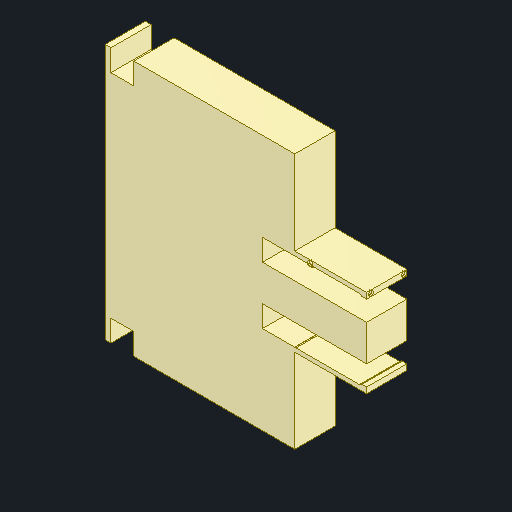
# Autodesk Inventor part: right_hold
Saved by Autodesk Inventor 2023 (Build 270158000, 158)
## iProperties
Created: 2024-05-18
Part Number: right_hold
Material: Nylon 6/6
Document SubType Name: Modeling
Designer: szymo
Density: 1.13 g/cm^3
Appearance: Nylon 6
Mass: 756.104 g
Surface Area: 779.57 cm^2
Volume: 669.119 cm^3
Author: szymo
Autodesk Inventor part; units mm, degrees
(part 1 of 2)
ref_plane "YZ Plane" through (0, 0, 0) normal (1, 0, 0) x (0, 1, 0)
ref_plane "XZ Plane" through (0, 0, 0) normal (0, 1, 0) x (-1, 0, 0)
ref_plane "XY Plane" through (0, 0, 0) normal (0, 0, 1) x (1, 0, 0)
ref_plane "Work Plane1" through (0, 0, 0) normal (0, 0, 1) x (1, 0, 0)
sketch "Sketch1" plane through (0, 0, 0) normal (0, 0, 1) x (1, 0, 0)
  line L0 (-71, -74) -> (-71, -89) projected
  line L1 (-71, -89) -> (41, -89) projected
  line L2 (41, -89) -> (41, -30.5) projected
  line L3 (41, -30.5) -> (91, -30.5) projected
  line L4 (91, -30.5) -> (91, -26.5) projected
  line L5 (91, 30.5) -> (41, 30.5) projected
  line L6 (41, 30.5) -> (41, 89) projected
  line L7 (41, 89) -> (-71, 89) projected
  line L8 (-71, 89) -> (-71, 74) projected
  line L9 (-71, 74) -> (-87, 74) projected
  line L10 (-87, 74) -> (-87, 89) projected
  line L11 (-87, 89) -> (-91, 89) projected
  line L12 (-91, 89) -> (-91, -89) projected
  line L13 (-91, -89) -> (-87, -89) projected
  line L14 (-87, -89) -> (-87, -74) projected
  line L15 (-87, -74) -> (-71, -74) projected
  line L16 (91, 30.5) -> (12, 30.5)
  line L17 (12, 30.5) -> (12, 29.5)
  line L18 (12, 29.5) -> (91, 29.5)
  line L19 (91, 29.5) -> (91, 30.5)
  line L20 (71.5, 26) -> (60.5, 26) projected
  line L21 (11.5, 37) -> (39.5, 37) projected
  line L22 (11, 8.5) -> (11, 9.5)
  circle A0 centre (15.25, 24.25) radius 1.8 projected
  circle A1 centre (15.25, -15.75) radius 1.8 projected
  circle A2 centre (6.1414, -28.5) radius 1.8 projected
  circle A3 centre (-23.4, 24.1) radius 1.8 projected
  circle A4 centre (-71.6, -24.1) radius 1.8 projected
  circle A5 centre (-82.75, 33.75) radius 1.8 projected
  circle A6 centre (-67.5, -84.5) radius 1.8 projected
  circle A7 centre (88, -10.5) radius 1.8 projected
  circle A8 centre (88, 10.5) radius 1.8 projected
  circle A9 centre (-67.5, 84.5) radius 1.8 projected
  circle A10 centre (-71.6, 24.1) radius 1.8 projected
  circle A11 centre (-82.75, -33.75) radius 1.8 projected
  circle A12 centre (-23.4, -24.1) radius 1.8 projected
  circle A13 centre (15.25, -24.25) radius 1.8 projected
  circle A14 centre (15.25, 15.75) radius 1.8 projected
  circle A15 centre (6.1414, 28.5) radius 1.8 projected
  circle A16 centre (-51.4385, -83.5) radius 1.55 projected
  circle A17 centre (-24.4119, -29.75) radius 1.55 projected
  circle A18 centre (-49.009, 29.75) radius 1.55 projected
  circle A19 centre (-22.5, 83.5) radius 1.55 projected
  circle A20 centre (8.5, -82.4087) radius 1.55 projected
  circle A21 centre (8.5, 82.4087) radius 1.55 projected
  circle A22 centre (-51.4385, 83.5) radius 1.55 projected
  circle A23 centre (-24.4119, 29.75) radius 1.55 projected
  circle A24 centre (-49.009, -29.75) radius 1.55 projected
  circle A25 centre (-22.5, -83.5) radius 1.55 projected
  circle A26 centre (-83, 21.5) radius 1.8 projected
  circle A27 centre (-83, -64.5) radius 1.8 projected
  circle A28 centre (-83, -21.5) radius 1.8 projected
  circle A29 centre (-83, 64.5) radius 1.8 projected
  line L23 (87.7321, 26.5) -> (91, 26.5) projected
  line L24 (91, 26.5) -> (91, 30.5) projected
  line L25 (91, -26.5) -> (87.7321, -26.5) projected
  arc A30 (87.7321, -26.5) -> (86.866, -27) centre (87.7321, -27.5) ccw projected
  arc A31 (86, -27.5) -> (86.866, -27) centre (86, -26.5) ccw projected
  line L26 (86, -27.5) -> (41.8217, -27.5) projected
  ellipse E0 centre (41.4293, -27.1664) end of major axis (40.558, -26.9979) minor radius 0.2933 (41, -27.3523) -> (41.8217, -27.5) ccw projected
  line L27 (41, -27.3523) -> (41, -27.5) projected
  line L28 (41, -27.5) -> (18.5, -27.5) projected
  line L29 (18.5, -27.5) -> (18.5, -12.5) projected
  line L30 (18.5, -12.5) -> (91, -12.5) projected
  line L31 (91, -12.5) -> (91, 12.5) projected
  line L32 (91, 12.5) -> (18.5, 12.5) projected
  line L33 (18.5, 12.5) -> (18.5, 27.5) projected
  line L34 (18.5, 27.5) -> (41, 27.5) projected
  line L35 (41, 27.5) -> (41, 27.3523) projected
  ellipse E1 centre (41.4293, 27.1664) end of major axis (40.558, 26.9979) minor radius 0.2933 (41.8217, 27.5) -> (41, 27.3523) ccw projected
  line L36 (41.8217, 27.5) -> (86, 27.5) projected
  arc A32 (86.866, 27) -> (86, 27.5) centre (86, 26.5) ccw projected
  arc A33 (86.866, 27) -> (87.7321, 26.5) centre (87.7321, 27.5) ccw projected
  line L37 (-85, 14) -> (-76, 14) projected
  line L38 (-76, 14) -> (-76, 20.1) projected
  line L39 (-76, 20.1) -> (11.5, 20.1) projected
  line L40 (11.5, 20.1) -> (11.5, 8.5) projected
  line L41 (11.5, 8.5) -> (84, 8.5) projected
  line L42 (84, 8.5) -> (84, -8.5) projected
  line L43 (84, -8.5) -> (11.5, -8.5) projected
  line L44 (11.5, -8.5) -> (11.5, -20.1) projected
  line L45 (11.5, -20.1) -> (-76, -20.1) projected
  line L46 (-76, -20.1) -> (-76, -14) projected
  line L47 (-76, -14) -> (-85, -14) projected
  arc A34 (-87, -12) -> (-85, -14) centre (-85, -12) ccw projected
  line L48 (-87, -12) -> (-87, 12) projected
  arc A35 (-85, 14) -> (-87, 12) centre (-85, 12) ccw projected
  line L49 (-76, 57) -> (-64, 69) projected
  line L50 (-64, 69) -> (-64, 79.9087) projected
  line L51 (-64, 79.9087) -> (15.1148, 79.9087) projected
  line L52 (15.1148, 79.9087) -> (15.1148, 37) projected
  line L53 (15.1148, 37) -> (-86, 37) projected
  line L54 (-86, 37) -> (-86, 29.2679) projected
  arc A36 (-87, 31) -> (-86, 29.2679) centre (-85, 31) ccw projected
  line L55 (-87, 31) -> (-87, 55) projected
  arc A37 (-85, 57) -> (-87, 55) centre (-85, 55) ccw projected
  line L56 (-85, 57) -> (-76, 57) projected
  line L57 (-64, -79.9087) -> (-64, -69) projected
  line L58 (-64, -69) -> (-76, -57) projected
  line L59 (-76, -57) -> (-85, -57) projected
  arc A38 (-87, -55) -> (-85, -57) centre (-85, -55) ccw projected
  line L60 (-87, -55) -> (-87, -37) projected
  line L61 (-87, -37) -> (15.1148, -37) projected
  line L62 (15.1148, -37) -> (15.1148, -79.9087) projected
  line L63 (15.1148, -79.9087) -> (-64, -79.9087) projected
  line L64 (30.8852, 37) -> (20.1148, 37) projected
  line L65 (20.1148, 37) -> (20.1148, 79.9087) projected
  line L66 (20.1148, 79.9087) -> (30.8852, 79.9087) projected
  line L67 (30.8852, 79.9087) -> (30.8852, 37) projected
  line L68 (30.8852, -79.9087) -> (20.1148, -79.9087) projected
  line L69 (20.1148, -79.9087) -> (20.1148, -37) projected
  line L70 (20.1148, -37) -> (30.8852, -37) projected
  line L71 (30.8852, -37) -> (30.8852, -79.9087) projected
  point P0 (0, 0)
  dimension "d0" = 0
  dimension "d1" = 3.5
  dimension "d2" = 1
  dimension "d14" = 1
  constraints: 10 end point, 2 parallel, 1 horizontal, 1 perpendicular, 1 point on line, 1 vertical, 4 other
  measures "d0" distance between parallel lines of L5 L16
  measures "d1" distance between parallel lines of L18 L20
  measures "d2" distance between parallel lines of L16 L18
  measures "d14" distance between parallel lines of L22 L17
ref_plane "Work Plane2" through (11, 8.5, 30) normal (0, 0, 1) x (1, 0, 0)
extrude "Extrusion1" add sketch "Sketch1" along normal blind 28 contours L15 L14 L13 L12 L11 L10 L9 L8 L7 L6 L16 L17 L18 L24 L23 A33 A32 L36 E1 L35 L34 L33 L32 L31 L30 L29 L28 L27 E0 L26 A31 A30 L25 L4 L3 L2 L1 L0 | L5 L19 L18 L17 L16 | L53 L54 A36 L55 A37 L56 L49 L50 L51 L52 L21 | L65 L66 L67 L21 | A0 | A1 | A2 | A3 | A4 | A5 | A6 | A7 | A8 | A9 | A10 | A11 | A12 | A13 | A14 | A15 | A16 | A17 | A18 | A19 | A20 | A21 | A22 | A23 | A24 | A25 | A26 | A27 | A28 | A29 | L37 L38 L39 L40 L41 L42 L43 L44 L45 L46 L47 A34 L48 A35 | L57 L58 L59 A38 L60 L61 L62 L63 | L68 L69 L70 L71
sketch "Sketch2" plane through (12, 29.5, 0) normal (0, -1, 0) x (1, 0, 0)
  circle A0 centre (54, 6.5) radius 3.9
  arc A1 (11.0575, 16.9943) -> (9.1437, 17.8944) centre (8.1132, 13.2185) ccw projected
  arc A2 (9.1437, 17.8944) -> (8.5881, 17.165) centre (13.5, 14) ccw projected
  arc A3 (8.5881, 17.165) -> (9.9644, 15.5591) centre (12.822, 19.4008) ccw projected
  arc A4 (9.9644, 15.5591) -> (9.764, 14.9868) centre (13.5, 14) ccw projected
  arc A5 (9.764, 14.9868) -> (7.6866, 14.59) centre (9.6013, 10.2015) ccw projected
  arc A6 (7.6866, 14.59) -> (7.6659, 13.6734) centre (13.5, 14) ccw projected
  arc A7 (7.6659, 13.6734) -> (9.7232, 13.1831) centre (9.777, 17.9709) ccw projected
  arc A8 (9.7232, 13.1831) -> (9.8975, 12.6024) centre (13.5, 14) ccw projected
  arc A9 (9.8975, 12.6024) -> (8.45, 11.0603) centre (12.5786, 8.6353) ccw projected
  arc A10 (8.45, 11.0603) -> (8.9721, 10.3065) centre (13.5, 14) ccw projected
  arc A11 (8.9721, 10.3065) -> (10.9247, 11.1192) centre (8.154, 15.0242) ccw projected
  arc A12 (10.9247, 11.1192) -> (11.407, 10.7518) centre (13.5, 14) ccw projected
  arc A13 (11.407, 10.7518) -> (11.1424, 8.6535) centre (15.9078, 9.1183) ccw projected
  arc A14 (11.1424, 8.6535) -> (12.0078, 8.3505) centre (13.5, 14) ccw projected
  arc A15 (12.0078, 8.3505) -> (13.1098, 10.1556) centre (8.573, 11.6863) ccw projected
  arc A16 (13.1098, 10.1556) -> (13.716, 10.1419) centre (13.5, 14) ccw projected
  arc A17 (13.716, 10.1419) -> (14.7353, 8.2888) centre (18.3174, 11.4659) ccw projected
  arc A18 (14.7353, 8.2888) -> (15.6135, 8.5523) centre (13.5, 14) ccw projected
  arc A19 (15.6135, 8.5523) -> (15.444, 10.6605) centre (10.8739, 9.2321) ccw projected
  arc A20 (15.444, 10.6605) -> (15.9425, 11.0057) centre (13.5, 14) ccw projected
  arc A21 (15.9425, 11.0057) -> (17.8563, 10.1056) centre (18.8868, 14.7815) ccw projected
  arc A22 (17.8563, 10.1056) -> (18.4119, 10.835) centre (13.5, 14) ccw projected
  arc A23 (18.4119, 10.835) -> (17.0356, 12.4409) centre (14.178, 8.5992) ccw projected
  arc A24 (17.0356, 12.4409) -> (17.236, 13.0132) centre (13.5, 14) ccw projected
  arc A25 (17.236, 13.0132) -> (19.3134, 13.41) centre (17.3987, 17.7985) ccw projected
  arc A26 (19.3134, 13.41) -> (19.3341, 14.3266) centre (13.5, 14) ccw projected
  arc A27 (19.3341, 14.3266) -> (17.2768, 14.8169) centre (17.223, 10.0291) ccw projected
  arc A28 (17.2768, 14.8169) -> (17.1025, 15.3976) centre (13.5, 14) ccw projected
  arc A29 (17.1025, 15.3976) -> (18.55, 16.9397) centre (14.4214, 19.3647) ccw projected
  arc A30 (18.55, 16.9397) -> (18.0279, 17.6935) centre (13.5, 14) ccw projected
  arc A31 (18.0279, 17.6935) -> (16.0753, 16.8808) centre (18.846, 12.9758) ccw projected
  arc A32 (16.0753, 16.8808) -> (15.593, 17.2482) centre (13.5, 14) ccw projected
  arc A33 (15.593, 17.2482) -> (15.8576, 19.3465) centre (11.0922, 18.8817) ccw projected
  arc A34 (15.8576, 19.3465) -> (14.9922, 19.6495) centre (13.5, 14) ccw projected
  arc A35 (14.9922, 19.6495) -> (13.8902, 17.8444) centre (18.427, 16.3137) ccw projected
  arc A36 (13.8902, 17.8444) -> (13.284, 17.8581) centre (13.5, 14) ccw projected
  arc A37 (13.284, 17.8581) -> (12.2647, 19.7112) centre (8.6826, 16.5341) ccw projected
  arc A38 (12.2647, 19.7112) -> (11.3865, 19.4477) centre (13.5, 14) ccw projected
  arc A39 (11.3865, 19.4477) -> (11.556, 17.3395) centre (16.1261, 18.7679) ccw projected
  arc A40 (11.556, 17.3395) -> (11.0575, 16.9943) centre (13.5, 14) ccw projected
  circle A41 centre (13.5, 14) radius 5.8433
  circle A42 centre (13.5, 14) radius 7
  circle A43 centre (54, 6.5) radius 3.5 projected
  point P0 (-12, 0)
  dimension "d12" = 11.6865
  dimension "d13" = 14
  dimension "d104" = 0.4
  constraints: 3 centre point, 3 coincident
  measures "d12" diameter of A41
  measures "d13" diameter of A42
  measures "d104" radial gap between concentric circles of A43 A0
extrude "Extrusion2" [suppressed]
sketch "Sketch3" plane through (12, 29.5, 0) normal (0, -1, 0) x (1, 0, 0)
  circle A0 centre (24.3093, 2.2034) radius 2 projected
  circle A1 centre (54, 6.5) radius 5.5 projected
  circle A2 centre (54, 6.5) radius 7.5
  circle A3 centre (24.3093, 2.2034) radius 4
  point P0 (-12, 0)
  dimension "d8" = 2
  dimension "d9" = 2
  constraints: 2 centre point
  measures "d8" radial gap between concentric circles of A1 A2
  measures "d9" radial gap between concentric circles of A0 A3
ref_plane "Work Plane3" through (58.3168, 26, -1.1832) normal (0, -1, 0) x (0.8086551, 0, -0.588283)
extrude "Extrusion3" [suppressed]
sketch "Sketch5" plane through (12, 29.5, 28) normal (0, -1, 0) x (1, 0, 0)
  spline S0 degree 3 poles (34.8142, -27.1484) (34.8967, -27.0725) (35.0616, -26.9208) (35.3204, -26.7061) (35.5433, -26.5363) (35.7266, -26.4074) (35.8666, -26.3142) (36.0095, -26.2258) (36.2022, -26.1113) (36.3834, -26.0337) (36.5239, -25.9411) (36.5769, -25.895) (36.615, -25.8538) (36.64, -25.82) (36.6627, -25.7845) (36.6816, -25.7469) (36.6965, -25.7076) (36.7072, -25.6669) (36.7147, -25.6254) (36.7153, -25.5834) (36.7146, -25.5413) (36.704, -25.4861) (36.6873, -25.4181) (36.6731, -25.3496) (36.6589, -25.2952) (36.6414, -25.2569) (36.6227, -25.2192) (36.5981, -25.185) (36.571, -25.1529) (36.5405, -25.1238) (36.5073, -25.098) (36.4716, -25.0758) (36.4344, -25.056) (36.3824, -25.0352) (36.3147, -25.0164) (36.1479, -24.9934) (35.951, -25.0013) (35.7278, -24.981) (35.5607, -24.9627) (35.3943, -24.9389) (35.1733, -24.9015) (34.899, -24.8441) (34.573, -24.7618) (34.3588, -24.6959) (34.2517, -24.6629) knots 0 0 0 0 0.033613 0.067227 0.100839 0.117647 0.134454 0.151261 0.168068 0.201677 0.210077 0.218473 0.222676 0.226878 0.231076 0.235279 0.239479 0.24368 0.247882 0.252083 0.256283 0.260485 0.268889 0.277292 0.281494 0.285694 0.289895 0.294097 0.298298 0.302498 0.306701 0.310899 0.315101 0.319304 0.3277 0.3361 0.369709 0.386516 0.403323 0.420131 0.436938 0.470551 0.504164 0.537777 0.537777 0.537777 0.537777 projected
  arc A0 (34.8142, -27.1484) -> (35.0416, -27.8703) centre (54, -21.5) ccw projected
  spline S1 degree 3 poles (36.0055, -30.2292) (36.0744, -30.1408) (36.2121, -29.964) (36.4321, -29.7097) (36.6239, -29.5054) (36.7836, -29.3481) (36.9063, -29.2332) (37.0327, -29.1225) (37.204, -28.9778) (37.3698, -28.8715) (37.4933, -28.757) (37.538, -28.7028) (37.5687, -28.6559) (37.5878, -28.6184) (37.6043, -28.5797) (37.6168, -28.5395) (37.625, -28.4983) (37.6289, -28.4564) (37.6294, -28.4142) (37.6231, -28.3726) (37.6155, -28.3312) (37.5959, -28.2786) (37.5684, -28.2142) (37.543, -28.149) (37.5201, -28.0977) (37.4965, -28.0628) (37.4719, -28.0287) (37.442, -27.999) (37.4099, -27.9718) (37.3751, -27.9481) (37.3381, -27.9281) (37.2992, -27.9121) (37.2593, -27.8987) (37.2045, -27.8867) (37.1347, -27.8794) (36.9664, -27.8841) (36.7735, -27.9243) (36.5499, -27.941) (36.3821, -27.9505) (36.2141, -27.9544) (35.9899, -27.9539) (35.71, -27.9425) (35.3748, -27.9149) (35.1527, -27.8851) (35.0416, -27.8703) knots 0 0 0 0 0.033613 0.067227 0.100839 0.117647 0.134454 0.151261 0.168068 0.201677 0.210077 0.218473 0.222676 0.226878 0.231076 0.235279 0.239479 0.24368 0.247882 0.252083 0.256283 0.260485 0.268889 0.277292 0.281494 0.285694 0.289895 0.294097 0.298298 0.302498 0.306701 0.310899 0.315101 0.319304 0.3277 0.3361 0.369709 0.386516 0.403323 0.420131 0.436938 0.470551 0.504164 0.537777 0.537777 0.537777 0.537777 projected
  arc A1 (36.0055, -30.2292) -> (36.3487, -30.9038) centre (54, -21.5) ccw projected
  spline S2 degree 3 poles (37.6878, -33.072) (37.7411, -32.9734) (37.8479, -32.7764) (38.0229, -32.4893) (38.1786, -32.2563) (38.3101, -32.0748) (38.4123, -31.9413) (38.5187, -31.8112) (38.6639, -31.6404) (38.81, -31.5082) (38.9129, -31.3749) (38.948, -31.3141) (38.9706, -31.2628) (38.9833, -31.2227) (38.9932, -31.1818) (38.9989, -31.1401) (39.0002, -31.098) (38.9972, -31.0561) (38.9907, -31.0144) (38.9777, -30.9744) (38.9633, -30.9349) (38.9354, -30.8861) (38.8976, -30.8272) (38.8618, -30.767) (38.8308, -30.7202) (38.8018, -30.6897) (38.7719, -30.6601) (38.7375, -30.6357) (38.7014, -30.6142) (38.6632, -30.5965) (38.6233, -30.5829) (38.5824, -30.5735) (38.5408, -30.5669) (38.4848, -30.5641) (38.4147, -30.5683) (38.2495, -30.6006) (38.0658, -30.6721) (37.8481, -30.7254) (37.6841, -30.7623) (37.519, -30.7938) (37.2979, -30.8302) (37.0198, -30.865) (36.6847, -30.893) (36.4607, -30.9002) (36.3487, -30.9038) knots 0 0 0 0 0.033613 0.067227 0.100839 0.117647 0.134454 0.151261 0.168068 0.201677 0.210077 0.218473 0.222676 0.226878 0.231076 0.235279 0.239479 0.24368 0.247882 0.252083 0.256283 0.260485 0.268889 0.277292 0.281494 0.285694 0.289895 0.294097 0.298298 0.302498 0.306701 0.310899 0.315101 0.319304 0.3277 0.3361 0.369709 0.386516 0.403323 0.420131 0.436938 0.470551 0.504164 0.537777 0.537777 0.537777 0.537777 projected
  arc A2 (37.6878, -33.072) -> (38.1373, -33.6809) centre (54, -21.5) ccw projected
  spline S3 degree 3 poles (39.8149, -35.5991) (39.8513, -35.4931) (39.9242, -35.2811) (40.0496, -34.9691) (40.1648, -34.7137) (40.2647, -34.5131) (40.3434, -34.3646) (40.427, -34.2187) (40.5421, -34.0263) (40.6644, -33.8719) (40.744, -33.7235) (40.7687, -33.6577) (40.7825, -33.6034) (40.7884, -33.5617) (40.7915, -33.5198) (40.7902, -33.4777) (40.7846, -33.436) (40.7747, -33.3952) (40.7615, -33.3551) (40.742, -33.3178) (40.7213, -33.2811) (40.6858, -33.2377) (40.6388, -33.1858) (40.5936, -33.1323) (40.5553, -33.0912) (40.5217, -33.0659) (40.4873, -33.0416) (40.4494, -33.0232) (40.4102, -33.0079) (40.3696, -32.9968) (40.3281, -32.9899) (40.2861, -32.9874) (40.244, -32.9877) (40.1883, -32.9942) (40.1198, -33.0099) (39.9622, -33.069) (39.7928, -33.1697) (39.5868, -33.2581) (39.4312, -33.3215) (39.2735, -33.3798) (39.0614, -33.452) (38.7928, -33.5321) (38.4669, -33.6149) (38.2471, -33.6589) (38.1373, -33.6809) knots 0 0 0 0 0.033613 0.067227 0.100839 0.117647 0.134454 0.151261 0.168068 0.201677 0.210077 0.218473 0.222676 0.226878 0.231076 0.235279 0.239479 0.24368 0.247882 0.252083 0.256283 0.260485 0.268889 0.277292 0.281494 0.285694 0.289895 0.294097 0.298298 0.302498 0.306701 0.310899 0.315101 0.319304 0.3277 0.3361 0.369709 0.386516 0.403323 0.420131 0.436938 0.470551 0.504164 0.537777 0.537777 0.537777 0.537777 projected
  arc A3 (39.8149, -35.5991) -> (40.3585, -36.1257) centre (54, -21.5) ccw projected
  spline S4 degree 3 poles (42.329, -37.7416) (42.3475, -37.631) (42.3845, -37.41) (42.4568, -37.0816) (42.5284, -36.8107) (42.5939, -36.5963) (42.6471, -36.4369) (42.7056, -36.2793) (42.7874, -36.0706) (42.8827, -35.8981) (42.9367, -35.7387) (42.9502, -35.6697) (42.9549, -35.6139) (42.9539, -35.5718) (42.95, -35.5299) (42.9418, -35.4886) (42.9294, -35.4484) (42.9129, -35.4097) (42.8933, -35.3724) (42.868, -35.3388) (42.8416, -35.306) (42.7993, -35.269) (42.7444, -35.2256) (42.6911, -35.1803) (42.6465, -35.1461) (42.6092, -35.1266) (42.5713, -35.1083) (42.5308, -35.0964) (42.4897, -35.0878) (42.4478, -35.0835) (42.4057, -35.0836) (42.3639, -35.088) (42.3224, -35.0952) (42.2686, -35.1107) (42.2036, -35.1375) (42.0578, -35.2217) (41.9074, -35.3489) (41.7187, -35.47) (41.5756, -35.5582) (41.4297, -35.6416) (41.2323, -35.7479) (40.9807, -35.8711) (40.6728, -36.0064) (40.4633, -36.0859) (40.3585, -36.1257) knots 0 0 0 0 0.033613 0.067227 0.100839 0.117647 0.134454 0.151261 0.168068 0.201677 0.210077 0.218473 0.222676 0.226878 0.231076 0.235279 0.239479 0.24368 0.247882 0.252083 0.256283 0.260485 0.268889 0.277292 0.281494 0.285694 0.289895 0.294097 0.298298 0.302498 0.306701 0.310899 0.315101 0.319304 0.3277 0.3361 0.369709 0.386516 0.403323 0.420131 0.436938 0.470551 0.504164 0.537777 0.537777 0.537777 0.537777 projected
  arc A4 (42.329, -37.7416) -> (42.9519, -38.1715) centre (54, -21.5) ccw projected
  spline S5 degree 3 poles (45.1615, -39.441) (45.1615, -39.329) (45.1616, -39.1048) (45.1789, -38.769) (45.2049, -38.49) (45.2342, -38.2678) (45.2605, -38.1018) (45.2922, -37.9367) (45.3386, -37.7174) (45.4041, -37.5316) (45.4312, -37.3654) (45.4332, -37.2952) (45.4286, -37.2393) (45.4207, -37.198) (45.41, -37.1573) (45.3951, -37.118) (45.3763, -37.0803) (45.3536, -37.0449) (45.3281, -37.0113) (45.2976, -36.9824) (45.2661, -36.9544) (45.2184, -36.9248) (45.1571, -36.891) (45.097, -36.8551) (45.0474, -36.8287) (45.0074, -36.8156) (44.967, -36.8038) (44.9251, -36.7987) (44.8831, -36.797) (44.8411, -36.7997) (44.7996, -36.8067) (44.7591, -36.8179) (44.7194, -36.8318) (44.6688, -36.856) (44.6092, -36.8931) (44.4792, -37.0002) (44.3518, -37.1504) (44.1856, -37.3009) (44.059, -37.4114) (43.9288, -37.5178) (43.7516, -37.655) (43.5236, -37.818) (43.2422, -38.0021) (43.0487, -38.115) (42.9519, -38.1715) knots 0 0 0 0 0.033613 0.067227 0.100839 0.117647 0.134454 0.151261 0.168068 0.201677 0.210077 0.218473 0.222676 0.226878 0.231076 0.235279 0.239479 0.24368 0.247882 0.252083 0.256283 0.260485 0.268889 0.277292 0.281494 0.285694 0.289895 0.294097 0.298298 0.302498 0.306701 0.310899 0.315101 0.319304 0.3277 0.3361 0.369709 0.386516 0.403323 0.420131 0.436938 0.470551 0.504164 0.537777 0.537777 0.537777 0.537777 projected
  arc A5 (45.1615, -39.441) -> (45.8466, -39.7626) centre (54, -21.5) ccw projected
  spline S6 degree 3 poles (48.235, -40.6511) (48.2166, -40.5406) (48.1798, -40.3195) (48.1416, -39.9854) (48.1213, -39.7059) (48.1137, -39.4819) (48.1123, -39.3138) (48.1164, -39.1458) (48.126, -38.9218) (48.1601, -38.7278) (48.1594, -38.5594) (48.1498, -38.4898) (48.1361, -38.4355) (48.1215, -38.396) (48.1043, -38.3577) (48.0831, -38.3213) (48.0583, -38.2872) (48.0301, -38.256) (47.9995, -38.2271) (47.9646, -38.2036) (47.929, -38.1811) (47.877, -38.1599) (47.811, -38.1366) (47.7458, -38.1111) (47.6925, -38.0932) (47.6509, -38.0869) (47.6091, -38.0819) (47.567, -38.0838) (47.5253, -38.089) (47.4843, -38.0985) (47.4445, -38.1122) (47.4064, -38.13) (47.3695, -38.1503) (47.3236, -38.1825) (47.2709, -38.2289) (47.1603, -38.3559) (47.0593, -38.525) (46.9202, -38.7008) (46.8135, -38.8307) (46.7026, -38.957) (46.5504, -39.1215) (46.3524, -39.3198) (46.1051, -39.5477) (45.9328, -39.691) (45.8466, -39.7626) knots 0 0 0 0 0.033613 0.067227 0.100839 0.117647 0.134454 0.151261 0.168068 0.201677 0.210077 0.218473 0.222676 0.226878 0.231076 0.235279 0.239479 0.24368 0.247882 0.252083 0.256283 0.260485 0.268889 0.277292 0.281494 0.285694 0.289895 0.294097 0.298298 0.302498 0.306701 0.310899 0.315101 0.319304 0.3277 0.3361 0.369709 0.386516 0.403323 0.420131 0.436938 0.470551 0.504164 0.537777 0.537777 0.537777 0.537777 projected
  arc A6 (48.235, -40.6511) -> (48.9637, -40.8555) centre (54, -21.5) ccw projected
  spline S7 degree 3 poles (51.4658, -41.3388) (51.4294, -41.2328) (51.3567, -41.0208) (51.2641, -40.6975) (51.1981, -40.4252) (51.1537, -40.2055) (51.1246, -40.04) (51.101, -39.8736) (51.0736, -39.6511) (51.0753, -39.454) (51.047, -39.2881) (51.0261, -39.221) (51.0036, -39.1696) (50.9827, -39.1331) (50.9593, -39.0982) (50.9325, -39.0657) (50.9024, -39.0363) (50.8695, -39.0101) (50.8345, -38.9866) (50.7962, -38.9692) (50.7574, -38.9529) (50.7026, -38.9405) (50.6337, -38.9283) (50.5652, -38.9139) (50.5097, -38.9051) (50.4676, -38.9057) (50.4256, -38.9076) (50.3843, -38.9164) (50.344, -38.9284) (50.3052, -38.9446) (50.2682, -38.9647) (50.2335, -38.9884) (50.2005, -39.0145) (50.1605, -39.0538) (50.1161, -39.1083) (50.028, -39.2517) (49.9562, -39.4352) (49.8479, -39.6315) (49.764, -39.7772) (49.6754, -39.92) (49.5524, -40.1073) (49.3897, -40.3355) (49.1834, -40.601) (49.0369, -40.7707) (48.9637, -40.8555) knots 0 0 0 0 0.033613 0.067227 0.100839 0.117647 0.134454 0.151261 0.168068 0.201677 0.210077 0.218473 0.222676 0.226878 0.231076 0.235279 0.239479 0.24368 0.247882 0.252083 0.256283 0.260485 0.268889 0.277292 0.281494 0.285694 0.289895 0.294097 0.298298 0.302498 0.306701 0.310899 0.315101 0.319304 0.3277 0.3361 0.369709 0.386516 0.403323 0.420131 0.436938 0.470551 0.504164 0.537777 0.537777 0.537777 0.537777 projected
  arc A7 (51.4658, -41.3388) -> (52.2182, -41.4205) centre (54, -21.5) ccw projected
  spline S8 degree 3 poles (54.7657, -41.4853) (54.7124, -41.3868) (54.6058, -41.1896) (54.4612, -40.886) (54.3513, -40.6283) (54.2713, -40.4189) (54.2154, -40.2604) (54.1648, -40.1001) (54.1011, -39.8852) (54.0704, -39.6905) (54.0151, -39.5315) (53.9834, -39.4688) (53.9528, -39.4218) (53.9262, -39.3893) (53.8974, -39.3586) (53.8656, -39.3311) (53.8311, -39.3069) (53.7943, -39.2866) (53.7559, -39.2692) (53.7153, -39.2582) (53.6743, -39.2486) (53.6182, -39.2453) (53.5482, -39.2447) (53.4783, -39.2418) (53.4221, -39.2422) (53.3807, -39.2497) (53.3395, -39.2586) (53.3003, -39.274) (53.2625, -39.2925) (53.2268, -39.3148) (53.1937, -39.3407) (53.1634, -39.3699) (53.1351, -39.401) (53.1021, -39.4464) (53.0673, -39.5074) (53.004, -39.6634) (52.9634, -39.8562) (52.8889, -40.0676) (52.8301, -40.2251) (52.7662, -40.3806) (52.6757, -40.5856) (52.5528, -40.8374) (52.393, -41.1333) (52.2765, -41.3247) (52.2182, -41.4205) knots 0 0 0 0 0.033613 0.067227 0.100839 0.117647 0.134454 0.151261 0.168068 0.201677 0.210077 0.218473 0.222676 0.226878 0.231076 0.235279 0.239479 0.24368 0.247882 0.252083 0.256283 0.260485 0.268889 0.277292 0.281494 0.285694 0.289895 0.294097 0.298298 0.302498 0.306701 0.310899 0.315101 0.319304 0.3277 0.3361 0.369709 0.386516 0.403323 0.420131 0.436938 0.470551 0.504164 0.537777 0.537777 0.537777 0.537777 projected
  arc A8 (54.7657, -41.4853) -> (55.5213, -41.4421) centre (54, -21.5) ccw projected
  spline S9 degree 3 poles (58.0448, -41.0867) (57.976, -40.9983) (57.8384, -40.8214) (57.6458, -40.5457) (57.4949, -40.3096) (57.3816, -40.1162) (57.3003, -39.9691) (57.224, -39.8193) (57.1258, -39.6178) (57.0635, -39.4309) (56.9828, -39.2831) (56.9412, -39.2265) (56.9033, -39.1852) (56.8716, -39.1574) (56.8382, -39.1319) (56.8023, -39.11) (56.7643, -39.0919) (56.7247, -39.0778) (56.6839, -39.067) (56.642, -39.0629) (56.6, -39.0601) (56.5442, -39.0661) (56.475, -39.0771) (56.4056, -39.0857) (56.3502, -39.0953) (56.3106, -39.1096) (56.2715, -39.1251) (56.2353, -39.1467) (56.2011, -39.1712) (56.1696, -39.1991) (56.1412, -39.2301) (56.1161, -39.2638) (56.0933, -39.2992) (56.0683, -39.3494) (56.044, -39.4153) (56.0072, -39.5796) (55.9989, -39.7765) (55.9602, -39.9973) (55.9281, -40.1623) (55.8907, -40.3262) (55.8352, -40.5433) (55.7554, -40.8119) (55.6464, -41.13) (55.563, -41.338) (55.5213, -41.4421) knots 0 0 0 0 0.033613 0.067227 0.100839 0.117647 0.134454 0.151261 0.168068 0.201677 0.210077 0.218473 0.222676 0.226878 0.231076 0.235279 0.239479 0.24368 0.247882 0.252083 0.256283 0.260485 0.268889 0.277292 0.281494 0.285694 0.289895 0.294097 0.298298 0.302498 0.306701 0.310899 0.315101 0.319304 0.3277 0.3361 0.369709 0.386516 0.403323 0.420131 0.436938 0.470551 0.504164 0.537777 0.537777 0.537777 0.537777 projected
  arc A9 (58.0448, -41.0867) -> (58.7829, -40.9197) centre (54, -21.5) ccw projected
  spline S10 degree 3 poles (61.2135, -40.1538) (61.131, -40.0779) (60.9662, -39.9261) (60.7309, -39.6859) (60.5432, -39.4778) (60.3996, -39.3057) (60.2952, -39.1739) (60.1953, -39.0388) (60.0653, -38.8562) (59.973, -38.6821) (59.8691, -38.5496) (59.8188, -38.5006) (59.7746, -38.4661) (59.7388, -38.444) (59.7016, -38.4243) (59.6626, -38.4086) (59.6221, -38.397) (59.5807, -38.3896) (59.5388, -38.3856) (59.4968, -38.3885) (59.4549, -38.3927) (59.4008, -38.4078) (59.3344, -38.43) (59.2673, -38.4499) (59.2143, -38.4685) (59.1775, -38.4891) (59.1415, -38.5108) (59.1094, -38.5381) (59.0797, -38.5679) (59.0532, -38.6006) (59.0302, -38.6359) (59.011, -38.6733) (58.9944, -38.7119) (58.978, -38.7655) (58.9648, -38.8345) (58.9556, -39.0026) (58.9798, -39.1982) (58.978, -39.4224) (58.9736, -39.5904) (58.9636, -39.7582) (58.9446, -39.9815) (58.9101, -40.2596) (58.855, -40.5913) (58.8069, -40.8102) (58.7829, -40.9197) knots 0 0 0 0 0.033613 0.067227 0.100839 0.117647 0.134454 0.151261 0.168068 0.201677 0.210077 0.218473 0.222676 0.226878 0.231076 0.235279 0.239479 0.24368 0.247882 0.252083 0.256283 0.260485 0.268889 0.277292 0.281494 0.285694 0.289895 0.294097 0.298298 0.302498 0.306701 0.310899 0.315101 0.319304 0.3277 0.3361 0.369709 0.386516 0.403323 0.420131 0.436938 0.470551 0.504164 0.537777 0.537777 0.537777 0.537777 projected
  arc A10 (61.2135, -40.1538) -> (61.9141, -39.8676) centre (54, -21.5) ccw projected
  spline S11 degree 3 poles (64.1854, -38.7121) (64.0916, -38.6508) (63.904, -38.5282) (63.6324, -38.33) (63.413, -38.1556) (63.243, -38.0095) (63.1184, -37.8967) (62.9976, -37.7799) (62.8393, -37.6211) (62.7196, -37.4646) (62.5953, -37.3511) (62.5376, -37.311) (62.4883, -37.2843) (62.4494, -37.2683) (62.4095, -37.255) (62.3684, -37.2459) (62.3266, -37.2411) (62.2845, -37.2407) (62.2425, -37.2437) (62.2016, -37.2534) (62.1609, -37.2644) (62.11, -37.2883) (62.0482, -37.3211) (61.9853, -37.3517) (61.9361, -37.3788) (61.9032, -37.4052) (61.8713, -37.4325) (61.8441, -37.4648) (61.8197, -37.499) (61.7989, -37.5356) (61.7821, -37.5742) (61.7693, -37.6143) (61.7593, -37.6551) (61.7519, -37.7107) (61.7503, -37.7809) (61.7689, -37.9483) (61.8249, -38.1372) (61.86, -38.3586) (61.8833, -38.525) (61.9011, -38.6922) (61.9191, -38.9156) (61.9308, -39.1955) (61.9311, -39.5318) (61.9197, -39.7557) (61.9141, -39.8676) knots 0 0 0 0 0.033613 0.067227 0.100839 0.117647 0.134454 0.151261 0.168068 0.201677 0.210077 0.218473 0.222676 0.226878 0.231076 0.235279 0.239479 0.24368 0.247882 0.252083 0.256283 0.260485 0.268889 0.277292 0.281494 0.285694 0.289895 0.294097 0.298298 0.302498 0.306701 0.310899 0.315101 0.319304 0.3277 0.3361 0.369709 0.386516 0.403323 0.420131 0.436938 0.470551 0.504164 0.537777 0.537777 0.537777 0.537777 projected
  arc A11 (64.1854, -38.7121) -> (64.8293, -38.3144) centre (54, -21.5) ccw projected
  spline S12 degree 3 poles (66.8795, -36.8009) (66.7769, -36.7559) (66.5717, -36.6658) (66.2711, -36.515) (66.0261, -36.3791) (65.8344, -36.263) (65.6929, -36.1723) (65.5545, -36.0769) (65.3722, -35.9464) (65.2284, -35.8117) (65.0871, -35.7201) (65.0236, -35.6901) (64.9706, -35.6718) (64.9295, -35.6625) (64.888, -35.656) (64.846, -35.6538) (64.8039, -35.6559) (64.7624, -35.6625) (64.7214, -35.6723) (64.6826, -35.6886) (64.6444, -35.7062) (64.5981, -35.7381) (64.5425, -35.7806) (64.4855, -35.8212) (64.4414, -35.856) (64.4134, -35.8874) (64.3863, -35.9197) (64.3649, -35.9559) (64.3464, -35.9937) (64.332, -36.0333) (64.3217, -36.0741) (64.3157, -36.1157) (64.3125, -36.1576) (64.3144, -36.2137) (64.3243, -36.2832) (64.3702, -36.4452) (64.4566, -36.6223) (64.5277, -36.8349) (64.578, -36.9953) (64.6231, -37.1572) (64.6776, -37.3746) (64.7353, -37.6488) (64.7908, -37.9805) (64.8165, -38.2031) (64.8293, -38.3144) knots 0 0 0 0 0.033613 0.067227 0.100839 0.117647 0.134454 0.151261 0.168068 0.201677 0.210077 0.218473 0.222676 0.226878 0.231076 0.235279 0.239479 0.24368 0.247882 0.252083 0.256283 0.260485 0.268889 0.277292 0.281494 0.285694 0.289895 0.294097 0.298298 0.302498 0.306701 0.310899 0.315101 0.319304 0.3277 0.3361 0.369709 0.386516 0.403323 0.420131 0.436938 0.470551 0.504164 0.537777 0.537777 0.537777 0.537777 projected
  arc A12 (66.8795, -36.8009) -> (67.4492, -36.3027) centre (54, -21.5) ccw projected
  spline S13 degree 3 poles (69.2223, -34.4723) (69.1137, -34.4448) (68.8964, -34.3897) (68.5751, -34.2904) (68.3111, -34.1968) (68.1029, -34.1138) (67.9484, -34.0476) (67.7961, -33.9763) (67.5949, -33.8775) (67.4309, -33.7684) (67.2764, -33.7013) (67.2089, -33.6822) (67.1536, -33.6729) (67.1116, -33.6704) (67.0695, -33.6708) (67.0277, -33.6756) (66.9866, -33.6846) (66.9467, -33.6979) (66.9079, -33.7143) (66.8723, -33.7368) (66.8374, -33.7604) (66.7971, -33.7995) (66.7492, -33.8506) (66.6997, -33.9) (66.6619, -33.9416) (66.6394, -33.9772) (66.6181, -34.0135) (66.6029, -34.0528) (66.5909, -34.0931) (66.5831, -34.1345) (66.5797, -34.1764) (66.5806, -34.2185) (66.5844, -34.2604) (66.5955, -34.3153) (66.6168, -34.3823) (66.6887, -34.5345) (66.803, -34.695) (66.9081, -34.893) (66.9842, -35.0429) (67.0553, -35.1952) (67.1448, -35.4006) (67.2469, -35.6616) (67.3563, -35.9796) (67.4182, -36.195) (67.4492, -36.3027) knots 0 0 0 0 0.033613 0.067227 0.100839 0.117647 0.134454 0.151261 0.168068 0.201677 0.210077 0.218473 0.222676 0.226878 0.231076 0.235279 0.239479 0.24368 0.247882 0.252083 0.256283 0.260485 0.268889 0.277292 0.281494 0.285694 0.289895 0.294097 0.298298 0.302498 0.306701 0.310899 0.315101 0.319304 0.3277 0.3361 0.369709 0.386516 0.403323 0.420131 0.436938 0.470551 0.504164 0.537777 0.537777 0.537777 0.537777 projected
  arc A13 (69.2223, -34.4723) -> (69.7022, -33.8871) centre (54, -21.5) ccw projected
  spline S14 degree 3 poles (71.1499, -31.7899) (71.0382, -31.7806) (70.8148, -31.762) (70.4816, -31.717) (70.2057, -31.6681) (69.9867, -31.6205) (69.8234, -31.5806) (69.6615, -31.5354) (69.4467, -31.4711) (69.267, -31.3904) (69.1036, -31.3497) (69.0338, -31.3419) (68.9777, -31.3418) (68.9359, -31.3463) (68.8945, -31.3536) (68.854, -31.3652) (68.815, -31.3809) (68.7778, -31.4006) (68.7422, -31.4232) (68.7108, -31.4512) (68.6804, -31.4802) (68.647, -31.5254) (68.6082, -31.5837) (68.5674, -31.6406) (68.537, -31.6878) (68.5207, -31.7267) (68.5056, -31.7659) (68.4971, -31.8072) (68.4919, -31.8489) (68.4911, -31.891) (68.4946, -31.933) (68.5025, -31.9743) (68.5131, -32.015) (68.533, -32.0674) (68.5651, -32.1299) (68.661, -32.2682) (68.8002, -32.4077) (68.9365, -32.5857) (69.0362, -32.721) (69.1314, -32.8596) (69.2535, -33.0475) (69.3971, -33.2881) (69.5574, -33.5837) (69.6539, -33.786) (69.7022, -33.8871) knots 0 0 0 0 0.033613 0.067227 0.100839 0.117647 0.134454 0.151261 0.168068 0.201677 0.210077 0.218473 0.222676 0.226878 0.231076 0.235279 0.239479 0.24368 0.247882 0.252083 0.256283 0.260485 0.268889 0.277292 0.281494 0.285694 0.289895 0.294097 0.298298 0.302498 0.306701 0.310899 0.315101 0.319304 0.3277 0.3361 0.369709 0.386516 0.403323 0.420131 0.436938 0.470551 0.504164 0.537777 0.537777 0.537777 0.537777 projected
  arc A14 (71.1499, -31.7899) -> (71.5269, -31.1337) centre (54, -21.5) ccw projected
  spline S15 degree 3 poles (72.6096, -28.8268) (72.4979, -28.836) (72.2746, -28.8544) (71.9385, -28.8649) (71.6583, -28.862) (71.4344, -28.8512) (71.2668, -28.8387) (71.0997, -28.8207) (70.8773, -28.7926) (70.6867, -28.7426) (70.5188, -28.7294) (70.4487, -28.7332) (70.3934, -28.7424) (70.3529, -28.7537) (70.3132, -28.7677) (70.2752, -28.7858) (70.2393, -28.8077) (70.2058, -28.8332) (70.1745, -28.8613) (70.1481, -28.8942) (70.1228, -28.9278) (70.0973, -28.9779) (70.0687, -29.0417) (70.0378, -29.1046) (70.0156, -29.1562) (70.0059, -29.1971) (69.9975, -29.2384) (69.9959, -29.2805) (69.9976, -29.3225) (70.0038, -29.3642) (70.0141, -29.4049) (70.0287, -29.4444) (70.0459, -29.4828) (70.0741, -29.5312) (70.116, -29.5876) (70.2335, -29.7082) (70.3937, -29.8229) (70.5574, -29.9761) (70.678, -30.0931) (70.7947, -30.2141) (70.9461, -30.3793) (71.1274, -30.5931) (71.3341, -30.8583) (71.4626, -31.0419) (71.5269, -31.1337) knots 0 0 0 0 0.033613 0.067227 0.100839 0.117647 0.134454 0.151261 0.168068 0.201677 0.210077 0.218473 0.222676 0.226878 0.231076 0.235279 0.239479 0.24368 0.247882 0.252083 0.256283 0.260485 0.268889 0.277292 0.281494 0.285694 0.289895 0.294097 0.298298 0.302498 0.306701 0.310899 0.315101 0.319304 0.3277 0.3361 0.369709 0.386516 0.403323 0.420131 0.436938 0.470551 0.504164 0.537777 0.537777 0.537777 0.537777 projected
  arc A15 (72.6096, -28.8268) -> (72.8735, -28.1174) centre (54, -21.5) ccw projected
  spline S16 degree 3 poles (73.5618, -25.6638) (73.4531, -25.6913) (73.2358, -25.7462) (72.906, -25.8119) (72.6292, -25.8552) (72.4066, -25.8813) (72.2392, -25.8966) (72.0714, -25.9063) (71.8474, -25.9153) (71.6512, -25.8973) (71.4835, -25.9119) (71.4149, -25.9272) (71.3618, -25.9453) (71.3237, -25.9631) (71.2869, -25.9835) (71.2524, -26.0076) (71.2206, -26.0351) (71.1918, -26.0658) (71.1655, -26.0987) (71.1449, -26.1354) (71.1255, -26.1728) (71.1086, -26.2263) (71.0908, -26.2941) (71.0708, -26.3611) (71.0574, -26.4157) (71.0545, -26.4577) (71.053, -26.4997) (71.0584, -26.5415) (71.067, -26.5827) (71.0799, -26.6228) (71.0968, -26.6613) (71.1177, -26.6978) (71.1409, -26.7329) (71.1768, -26.776) (71.2274, -26.8247) (71.3631, -26.9243) (71.54, -27.0111) (71.7267, -27.1352) (71.8649, -27.2308) (72, -27.3309) (72.1765, -27.469) (72.3904, -27.65) (72.638, -27.8775) (72.795, -28.0375) (72.8735, -28.1174) knots 0 0 0 0 0.033613 0.067227 0.100839 0.117647 0.134454 0.151261 0.168068 0.201677 0.210077 0.218473 0.222676 0.226878 0.231076 0.235279 0.239479 0.24368 0.247882 0.252083 0.256283 0.260485 0.268889 0.277292 0.281494 0.285694 0.289895 0.294097 0.298298 0.302498 0.306701 0.310899 0.315101 0.319304 0.3277 0.3361 0.369709 0.386516 0.403323 0.420131 0.436938 0.470551 0.504164 0.537777 0.537777 0.537777 0.537777 projected
  arc A16 (73.5618, -25.6638) -> (73.7053, -24.9207) centre (54, -21.5) ccw projected
  spline S17 degree 3 poles (73.9803, -22.3873) (73.8777, -22.4323) (73.6724, -22.5222) (73.3579, -22.6412) (73.092, -22.7295) (72.8767, -22.7919) (72.7141, -22.8345) (72.5502, -22.8718) (72.3307, -22.9175) (72.1342, -22.932) (71.9712, -22.974) (71.9061, -23.0004) (71.8567, -23.027) (71.8221, -23.0509) (71.7891, -23.077) (71.7591, -23.1065) (71.7322, -23.1388) (71.7088, -23.1738) (71.6883, -23.2106) (71.6741, -23.2502) (71.6611, -23.2903) (71.6532, -23.3459) (71.6468, -23.4156) (71.6381, -23.4851) (71.6338, -23.5411) (71.6379, -23.583) (71.6434, -23.6247) (71.6555, -23.6651) (71.6708, -23.7042) (71.6901, -23.7416) (71.7132, -23.7768) (71.7397, -23.8095) (71.7685, -23.8402) (71.8109, -23.8768) (71.8689, -23.9165) (72.0191, -23.9925) (72.2079, -24.0489) (72.4125, -24.1406) (72.5645, -24.2122) (72.7142, -24.2887) (72.9111, -24.3958) (73.1519, -24.5391) (73.4335, -24.7228) (73.6147, -24.8548) (73.7053, -24.9207) knots 0 0 0 0 0.033613 0.067227 0.100839 0.117647 0.134454 0.151261 0.168068 0.201677 0.210077 0.218473 0.222676 0.226878 0.231076 0.235279 0.239479 0.24368 0.247882 0.252083 0.256283 0.260485 0.268889 0.277292 0.281494 0.285694 0.289895 0.294097 0.298298 0.302498 0.306701 0.310899 0.315101 0.319304 0.3277 0.3361 0.369709 0.386516 0.403323 0.420131 0.436938 0.470551 0.504164 0.537777 0.537777 0.537777 0.537777 projected
  arc A17 (73.9803, -22.3873) -> (73.9996, -21.6307) centre (54, -21.5) ccw projected
  spline S18 degree 3 poles (73.8538, -19.0865) (73.76, -19.1478) (73.5723, -19.2703) (73.2817, -19.4395) (73.0339, -19.5703) (72.8319, -19.6673) (72.6785, -19.7361) (72.523, -19.7998) (72.314, -19.881) (72.1226, -19.9277) (71.9687, -19.9959) (71.9088, -20.0327) (71.8645, -20.0671) (71.8343, -20.0963) (71.8061, -20.1275) (71.7813, -20.1615) (71.7601, -20.1979) (71.7428, -20.2362) (71.7286, -20.2759) (71.7211, -20.3173) (71.7149, -20.359) (71.7162, -20.4151) (71.7214, -20.4849) (71.7242, -20.5549) (71.7293, -20.6108) (71.7402, -20.6515) (71.7524, -20.6917) (71.7711, -20.7295) (71.7926, -20.7657) (71.8178, -20.7994) (71.8463, -20.8303) (71.8779, -20.8581) (71.9113, -20.8837) (71.9592, -20.9128) (72.0229, -20.9425) (72.1836, -20.9927) (72.3791, -21.0172) (72.596, -21.074) (72.7578, -21.1196) (72.918, -21.1704) (73.1298, -21.2437) (73.3909, -21.3454) (73.6989, -21.4802) (73.8994, -21.5805) (73.9996, -21.6307) knots 0 0 0 0 0.033613 0.067227 0.100839 0.117647 0.134454 0.151261 0.168068 0.201677 0.210077 0.218473 0.222676 0.226878 0.231076 0.235279 0.239479 0.24368 0.247882 0.252083 0.256283 0.260485 0.268889 0.277292 0.281494 0.285694 0.289895 0.294097 0.298298 0.302498 0.306701 0.310899 0.315101 0.319304 0.3277 0.3361 0.369709 0.386516 0.403323 0.420131 0.436938 0.470551 0.504164 0.537777 0.537777 0.537777 0.537777 projected
  arc A18 (73.8538, -19.0865) -> (73.7483, -18.3371) centre (54, -21.5) ccw projected
  spline S19 degree 3 poles (73.1858, -15.8516) (73.1033, -15.9275) (72.9384, -16.0792) (72.6796, -16.2939) (72.4567, -16.4637) (72.2734, -16.5926) (72.1334, -16.6858) (71.9905, -16.7742) (71.7978, -16.8887) (71.6166, -16.9663) (71.4761, -17.0589) (71.4231, -17.105) (71.385, -17.1462) (71.36, -17.18) (71.3373, -17.2155) (71.3184, -17.2531) (71.3035, -17.2924) (71.2928, -17.3331) (71.2853, -17.3746) (71.2847, -17.4166) (71.2854, -17.4587) (71.296, -17.5139) (71.3127, -17.5819) (71.3269, -17.6504) (71.3411, -17.7048) (71.3586, -17.7431) (71.3773, -17.7808) (71.4019, -17.815) (71.429, -17.8471) (71.4595, -17.8762) (71.4927, -17.902) (71.5284, -17.9242) (71.5656, -17.944) (71.6176, -17.9648) (71.6853, -17.9836) (71.8521, -18.0066) (72.049, -17.9987) (72.2722, -18.019) (72.4393, -18.0373) (72.6057, -18.0611) (72.8267, -18.0985) (73.101, -18.1559) (73.427, -18.2382) (73.6412, -18.3041) (73.7483, -18.3371) knots 0 0 0 0 0.033613 0.067227 0.100839 0.117647 0.134454 0.151261 0.168068 0.201677 0.210077 0.218473 0.222676 0.226878 0.231076 0.235279 0.239479 0.24368 0.247882 0.252083 0.256283 0.260485 0.268889 0.277292 0.281494 0.285694 0.289895 0.294097 0.298298 0.302498 0.306701 0.310899 0.315101 0.319304 0.3277 0.3361 0.369709 0.386516 0.403323 0.420131 0.436938 0.470551 0.504164 0.537777 0.537777 0.537777 0.537777 projected
  arc A19 (73.1858, -15.8516) -> (72.9584, -15.1297) centre (54, -21.5) ccw projected
  spline S20 degree 3 poles (71.9945, -12.7708) (71.9256, -12.8592) (71.7879, -13.036) (71.5679, -13.2903) (71.3761, -13.4946) (71.2164, -13.6519) (71.0937, -13.7668) (70.9673, -13.8775) (70.796, -14.0222) (70.6302, -14.1285) (70.5067, -14.243) (70.462, -14.2972) (70.4313, -14.3441) (70.4122, -14.3816) (70.3957, -14.4203) (70.3832, -14.4605) (70.375, -14.5017) (70.3711, -14.5436) (70.3706, -14.5858) (70.3769, -14.6274) (70.3845, -14.6688) (70.4041, -14.7214) (70.4316, -14.7858) (70.457, -14.851) (70.4799, -14.9023) (70.5035, -14.9372) (70.5281, -14.9713) (70.558, -15.001) (70.5901, -15.0282) (70.6249, -15.0519) (70.6619, -15.0719) (70.7008, -15.0879) (70.7407, -15.1013) (70.7955, -15.1133) (70.8653, -15.1206) (71.0336, -15.1159) (71.2265, -15.0757) (71.4501, -15.059) (71.6179, -15.0495) (71.7859, -15.0456) (72.0101, -15.0461) (72.29, -15.0575) (72.6252, -15.0851) (72.8473, -15.1149) (72.9584, -15.1297) knots 0 0 0 0 0.033613 0.067227 0.100839 0.117647 0.134454 0.151261 0.168068 0.201677 0.210077 0.218473 0.222676 0.226878 0.231076 0.235279 0.239479 0.24368 0.247882 0.252083 0.256283 0.260485 0.268889 0.277292 0.281494 0.285694 0.289895 0.294097 0.298298 0.302498 0.306701 0.310899 0.315101 0.319304 0.3277 0.3361 0.369709 0.386516 0.403323 0.420131 0.436938 0.470551 0.504164 0.537777 0.537777 0.537777 0.537777 projected
  arc A20 (71.9945, -12.7708) -> (71.6513, -12.0962) centre (54, -21.5) ccw projected
  spline S21 degree 3 poles (70.3122, -9.928) (70.2589, -10.0266) (70.1521, -10.2236) (69.9771, -10.5107) (69.8214, -10.7437) (69.6899, -10.9252) (69.5877, -11.0587) (69.4813, -11.1888) (69.3361, -11.3596) (69.19, -11.4918) (69.0871, -11.6251) (69.052, -11.6859) (69.0294, -11.7372) (69.0167, -11.7773) (69.0068, -11.8182) (69.0011, -11.8599) (68.9998, -11.902) (69.0028, -11.9439) (69.0093, -11.9856) (69.0223, -12.0256) (69.0367, -12.0651) (69.0646, -12.1139) (69.1024, -12.1728) (69.1382, -12.233) (69.1692, -12.2798) (69.1982, -12.3103) (69.2281, -12.3399) (69.2625, -12.3643) (69.2986, -12.3858) (69.3368, -12.4035) (69.3767, -12.4171) (69.4176, -12.4265) (69.4592, -12.4331) (69.5152, -12.4359) (69.5853, -12.4317) (69.7505, -12.3994) (69.9342, -12.3279) (70.1519, -12.2746) (70.3159, -12.2377) (70.481, -12.2062) (70.7021, -12.1698) (70.9802, -12.135) (71.3153, -12.107) (71.5393, -12.0998) (71.6513, -12.0962) knots 0 0 0 0 0.033613 0.067227 0.100839 0.117647 0.134454 0.151261 0.168068 0.201677 0.210077 0.218473 0.222676 0.226878 0.231076 0.235279 0.239479 0.24368 0.247882 0.252083 0.256283 0.260485 0.268889 0.277292 0.281494 0.285694 0.289895 0.294097 0.298298 0.302498 0.306701 0.310899 0.315101 0.319304 0.3277 0.3361 0.369709 0.386516 0.403323 0.420131 0.436938 0.470551 0.504164 0.537777 0.537777 0.537777 0.537777 projected
  arc A21 (70.3122, -9.928) -> (69.8627, -9.3191) centre (54, -21.5) ccw projected
  spline S22 degree 3 poles (68.1851, -7.4009) (68.1487, -7.5069) (68.0758, -7.7189) (67.9504, -8.0309) (67.8352, -8.2863) (67.7353, -8.4869) (67.6566, -8.6354) (67.573, -8.7813) (67.4579, -8.9737) (67.3356, -9.1281) (67.256, -9.2765) (67.2313, -9.3423) (67.2175, -9.3966) (67.2116, -9.4383) (67.2085, -9.4802) (67.2098, -9.5223) (67.2154, -9.564) (67.2253, -9.6048) (67.2385, -9.6449) (67.258, -9.6822) (67.2787, -9.7189) (67.3142, -9.7623) (67.3612, -9.8142) (67.4064, -9.8677) (67.4447, -9.9088) (67.4783, -9.9341) (67.5127, -9.9584) (67.5506, -9.9768) (67.5898, -9.9921) (67.6304, -10.0032) (67.6719, -10.0101) (67.7139, -10.0126) (67.756, -10.0123) (67.8117, -10.0058) (67.8802, -9.9901) (68.0378, -9.931) (68.2072, -9.8303) (68.4132, -9.7419) (68.5688, -9.6785) (68.7265, -9.6202) (68.9386, -9.548) (69.2072, -9.4679) (69.5331, -9.3851) (69.7529, -9.3411) (69.8627, -9.3191) knots 0 0 0 0 0.033613 0.067227 0.100839 0.117647 0.134454 0.151261 0.168068 0.201677 0.210077 0.218473 0.222676 0.226878 0.231076 0.235279 0.239479 0.24368 0.247882 0.252083 0.256283 0.260485 0.268889 0.277292 0.281494 0.285694 0.289895 0.294097 0.298298 0.302498 0.306701 0.310899 0.315101 0.319304 0.3277 0.3361 0.369709 0.386516 0.403323 0.420131 0.436938 0.470551 0.504164 0.537777 0.537777 0.537777 0.537777 projected
  arc A22 (68.1851, -7.4009) -> (67.6415, -6.8743) centre (54, -21.5) ccw projected
  spline S23 degree 3 poles (65.671, -5.2584) (65.6525, -5.369) (65.6155, -5.59) (65.5432, -5.9184) (65.4716, -6.1893) (65.4061, -6.4037) (65.3529, -6.5631) (65.2944, -6.7207) (65.2126, -6.9294) (65.1173, -7.1019) (65.0633, -7.2613) (65.0498, -7.3303) (65.0451, -7.3861) (65.0461, -7.4282) (65.05, -7.4701) (65.0582, -7.5114) (65.0706, -7.5516) (65.0871, -7.5903) (65.1067, -7.6276) (65.132, -7.6612) (65.1584, -7.694) (65.2007, -7.731) (65.2556, -7.7744) (65.3089, -7.8197) (65.3535, -7.8539) (65.3908, -7.8734) (65.4287, -7.8917) (65.4692, -7.9036) (65.5103, -7.9122) (65.5522, -7.9165) (65.5943, -7.9164) (65.6361, -7.912) (65.6776, -7.9048) (65.7314, -7.8893) (65.7964, -7.8625) (65.9422, -7.7783) (66.0926, -7.6511) (66.2813, -7.53) (66.4244, -7.4418) (66.5703, -7.3584) (66.7677, -7.2521) (67.0193, -7.1289) (67.3272, -6.9936) (67.5367, -6.9141) (67.6415, -6.8743) knots 0 0 0 0 0.033613 0.067227 0.100839 0.117647 0.134454 0.151261 0.168068 0.201677 0.210077 0.218473 0.222676 0.226878 0.231076 0.235279 0.239479 0.24368 0.247882 0.252083 0.256283 0.260485 0.268889 0.277292 0.281494 0.285694 0.289895 0.294097 0.298298 0.302498 0.306701 0.310899 0.315101 0.319304 0.3277 0.3361 0.369709 0.386516 0.403323 0.420131 0.436938 0.470551 0.504164 0.537777 0.537777 0.537777 0.537777 projected
  arc A23 (65.671, -5.2584) -> (65.0481, -4.8285) centre (54, -21.5) ccw projected
  spline S24 degree 3 poles (62.8385, -3.559) (62.8385, -3.671) (62.8384, -3.8952) (62.8211, -4.231) (62.7951, -4.51) (62.7658, -4.7322) (62.7395, -4.8982) (62.7078, -5.0633) (62.6614, -5.2826) (62.5959, -5.4684) (62.5688, -5.6346) (62.5668, -5.7048) (62.5714, -5.7607) (62.5793, -5.802) (62.59, -5.8427) (62.6049, -5.882) (62.6237, -5.9197) (62.6464, -5.9551) (62.6719, -5.9887) (62.7024, -6.0176) (62.7339, -6.0456) (62.7816, -6.0752) (62.8429, -6.109) (62.903, -6.1449) (62.9526, -6.1713) (62.9926, -6.1844) (63.033, -6.1962) (63.0749, -6.2013) (63.1169, -6.203) (63.1589, -6.2003) (63.2004, -6.1933) (63.2409, -6.1821) (63.2806, -6.1682) (63.3312, -6.144) (63.3908, -6.1069) (63.5208, -5.9998) (63.6482, -5.8496) (63.8144, -5.6991) (63.941, -5.5886) (64.0712, -5.4822) (64.2484, -5.345) (64.4764, -5.182) (64.7578, -4.9979) (64.9513, -4.885) (65.0481, -4.8285) knots 0 0 0 0 0.033613 0.067227 0.100839 0.117647 0.134454 0.151261 0.168068 0.201677 0.210077 0.218473 0.222676 0.226878 0.231076 0.235279 0.239479 0.24368 0.247882 0.252083 0.256283 0.260485 0.268889 0.277292 0.281494 0.285694 0.289895 0.294097 0.298298 0.302498 0.306701 0.310899 0.315101 0.319304 0.3277 0.3361 0.369709 0.386516 0.403323 0.420131 0.436938 0.470551 0.504164 0.537777 0.537777 0.537777 0.537777 projected
  arc A24 (62.8385, -3.559) -> (62.1534, -3.2374) centre (54, -21.5) ccw projected
  spline S25 degree 3 poles (59.765, -2.3489) (59.7834, -2.4594) (59.8202, -2.6805) (59.8584, -3.0146) (59.8787, -3.2941) (59.8863, -3.5181) (59.8877, -3.6862) (59.8836, -3.8542) (59.874, -4.0782) (59.8399, -4.2722) (59.8406, -4.4406) (59.8502, -4.5102) (59.8639, -4.5645) (59.8785, -4.604) (59.8957, -4.6423) (59.9169, -4.6787) (59.9417, -4.7128) (59.9699, -4.744) (60.0005, -4.7729) (60.0354, -4.7964) (60.071, -4.8189) (60.123, -4.8401) (60.189, -4.8634) (60.2542, -4.8889) (60.3075, -4.9068) (60.3491, -4.9131) (60.3909, -4.9181) (60.433, -4.9162) (60.4747, -4.911) (60.5157, -4.9015) (60.5555, -4.8878) (60.5936, -4.87) (60.6305, -4.8497) (60.6764, -4.8175) (60.7291, -4.7711) (60.8397, -4.6441) (60.9407, -4.475) (61.0798, -4.2992) (61.1865, -4.1693) (61.2974, -4.043) (61.4496, -3.8785) (61.6476, -3.6802) (61.8949, -3.4523) (62.0672, -3.309) (62.1534, -3.2374) knots 0 0 0 0 0.033613 0.067227 0.100839 0.117647 0.134454 0.151261 0.168068 0.201677 0.210077 0.218473 0.222676 0.226878 0.231076 0.235279 0.239479 0.24368 0.247882 0.252083 0.256283 0.260485 0.268889 0.277292 0.281494 0.285694 0.289895 0.294097 0.298298 0.302498 0.306701 0.310899 0.315101 0.319304 0.3277 0.3361 0.369709 0.386516 0.403323 0.420131 0.436938 0.470551 0.504164 0.537777 0.537777 0.537777 0.537777 projected
  arc A25 (59.765, -2.3489) -> (59.0363, -2.1445) centre (54, -21.5) ccw projected
  spline S26 degree 3 poles (56.5342, -1.6612) (56.5706, -1.7672) (56.6433, -1.9792) (56.7359, -2.3025) (56.8019, -2.5748) (56.8463, -2.7945) (56.8754, -2.96) (56.899, -3.1264) (56.9264, -3.3489) (56.9247, -3.546) (56.953, -3.7119) (56.9739, -3.779) (56.9964, -3.8304) (57.0173, -3.8669) (57.0407, -3.9018) (57.0675, -3.9343) (57.0976, -3.9637) (57.1305, -3.9899) (57.1655, -4.0134) (57.2038, -4.0308) (57.2426, -4.0471) (57.2974, -4.0595) (57.3663, -4.0717) (57.4348, -4.0861) (57.4903, -4.0949) (57.5324, -4.0943) (57.5744, -4.0924) (57.6157, -4.0836) (57.656, -4.0716) (57.6948, -4.0554) (57.7318, -4.0353) (57.7665, -4.0116) (57.7995, -3.9855) (57.8395, -3.9462) (57.8839, -3.8917) (57.972, -3.7483) (58.0438, -3.5648) (58.1521, -3.3685) (58.236, -3.2228) (58.3246, -3.08) (58.4476, -2.8927) (58.6103, -2.6645) (58.8166, -2.399) (58.9631, -2.2293) (59.0363, -2.1445) knots 0 0 0 0 0.033613 0.067227 0.100839 0.117647 0.134454 0.151261 0.168068 0.201677 0.210077 0.218473 0.222676 0.226878 0.231076 0.235279 0.239479 0.24368 0.247882 0.252083 0.256283 0.260485 0.268889 0.277292 0.281494 0.285694 0.289895 0.294097 0.298298 0.302498 0.306701 0.310899 0.315101 0.319304 0.3277 0.3361 0.369709 0.386516 0.403323 0.420131 0.436938 0.470551 0.504164 0.537777 0.537777 0.537777 0.537777 projected
  arc A26 (56.5342, -1.6612) -> (55.7818, -1.5795) centre (54, -21.5) ccw projected